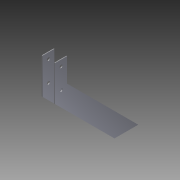
# Autodesk Inventor part: electronics board support
Saved by Autodesk Inventor 2012 (Build 160160000, 160)
## iProperties
Created: 2013-10-02
Part Number: electronics board support
Material: Default
Document SubType Name: Modeling
Designer: Bryce
Density: 1 g/cm^3
Author: Bryce
Autodesk Inventor part; units mm, degrees
ref_plane "YZ Plane" through (0, 0, 0) normal (1, 0, 0) x (0, 1, 0)
ref_plane "XZ Plane" through (0, 0, 0) normal (0, 1, 0) x (-1, 0, 0)
ref_plane "XY Plane" through (0, 0, 0) normal (0, 0, 1) x (1, 0, 0)
sketch "Sketch1" plane through (0, 0, 0) normal (0, 0, 1) x (1, 0, 0)
  line L0 (0, 0) -> (28.575, 0)
  line L1 (28.575, 0) -> (28.575, 203.2)
  line L2 (0, 203.2) -> (0, 0)
  line L3 (26.9875, 203.2) -> (26.9875, 1.5875)
  line L4 (26.9875, 1.5875) -> (1.5875, 1.5875)
  line L5 (1.5875, 1.5875) -> (1.5875, 203.2)
  line L6 (28.575, 203.2) -> (26.9875, 203.2)
  line L7 (1.5875, 203.2) -> (0, 203.2)
  dimension "d0" = 28.575
  dimension "d1" = 203.2
  dimension "d2" = 1.5875
  dimension "d3" = 1.5875
  dimension "d4" = 1.5875
  constraints: 16 end point, 4 parallel, 1 collinear, 1 horizontal, 1 perpendicular
  measures "d0" distance of L0.start L0.end
  measures "d1" distance of L2.start L0.start
  measures "d2" distance between parallel lines of L5 L2
  measures "d3" distance between parallel lines of L0 L4
  measures "d4" distance between parallel lines of L1 L3
extrude "Extrusion1" add sketch "Sketch1" along normal blind 177.8
sketch "Sketch2" plane through (28.575, 0, 0) normal (1, 0, 0) x (0, 0, -1)
  line L0 (-177.8, 203.2) -> (-177.8, 0) projected
  line L1 (0, 0) -> (-177.8, 0) projected
  line L2 (0, 0) -> (0, 203.2) projected
  line L3 (0, 203.2) -> (-177.8, 203.2) projected
  line L4 (-177.8, 127) -> (-50.8, 0)
  line L5 (0, 0) -> (-152.4, 152.4)
  line L6 (-152.4, 152.4) -> (-152.4, 203.2)
  circle A0 centre (-165.1, 146.5072) radius 3.175
  circle A1 centre (-165.1, 190.5) radius 3.175
  dimension "d7" = 50.8
  dimension "d8" = 45
  dimension "d9" = 25.4
  dimension "d10" = 6.35
  dimension "d11" = 12.7
  dimension "d12" = 12.7
  dimension "d13" = 43.9928
  constraints: 6 end point, 3 point on line, 2 centre point, 1 equal radius, 1 parallel, 1 perpendicular, 1 vertical alignment
  measures "d7" distance of L1.start L4.end
  measures "d8" angle of L1 L4
  measures "d9" distance between parallel lines of L0 L6
  measures "d10" diameter of A0
  measures "d11" distance from line of L0 A1.centre
  measures "d12" distance from line of L3 A1.centre
  measures "d13" distance of A0.centre A1.centre
extrude "Extrusion2" cut sketch "Sketch2" against normal blind 203.2 contours L4 L1 L0 | L3 L2 L5 L6 | A0 | A1
equation "\"d3\" = d2"
equation "\"d4\" = d3"
equation "\"d11\" = 0.5 * d9"
equation "\"d12\" = d11"
body "Solid1"
